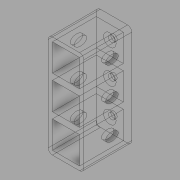
# Autodesk Inventor part: AK-C-C39-Holder
Saved by Autodesk Inventor 2016 (Build 200138000, 138)
## iProperties
Created: 2016-04-02
Part Number: AK-C-C39-Holder
Material: ABS Plastic
Document SubType Name: Modeling
Designer: admin
Density: 1.06 g/cm^3
Appearance: Smooth - White
Author: admin
Autodesk Inventor part; units mm, degrees
ref_plane "YZ Plane" through (0, 0, 0) normal (1, 0, 0) x (0, 1, 0)
ref_plane "XZ Plane" through (0, 0, 0) normal (0, 1, 0) x (-1, 0, 0)
ref_plane "XY Plane" through (0, 0, 0) normal (0, 0, 1) x (1, 0, 0)
derived "AK-C-C39-Main-Board.ipt"
sketch "Sketch2" plane through (0, 0, 0) normal (0, 1, 0) x (-1, 0, 0)
  line L0 (51.25, -29) -> (44.125, -29)
  line L1 (43.25, -29.875) -> (43.25, -31)
  line L2 (43.25, -31) -> (6.5, -31)
  line L3 (6.5, -31) -> (6.5, -29.875)
  line L4 (5.625, -29) -> (-5.625, -29)
  line L5 (-6.5, -29.875) -> (-6.5, -31)
  line L6 (-6.5, -31) -> (-43.25, -31)
  line L7 (-43.25, -31) -> (-43.25, -29.875)
  line L8 (-44.125, -29) -> (-51.25, -29)
  line L9 (-51.25, -29) -> (-53.75, -26.5)
  line L10 (-53.75, -26.5) -> (-53.75, 26.5)
  line L11 (-53.75, 26.5) -> (-51.25, 29)
  line L12 (-51.25, 29) -> (-44.125, 29)
  line L13 (-43.25, 29.875) -> (-43.25, 31)
  line L14 (-43.25, 31) -> (-6.5, 31)
  line L15 (-6.5, 31) -> (-6.5, 29.875)
  line L16 (-5.625, 29) -> (5.625, 29)
  line L17 (6.5, 29.875) -> (6.5, 31)
  line L18 (43.25, 31) -> (43.25, 29.875)
  line L19 (43.25, 31) -> (6.5, 31)
  line L20 (44.125, 29) -> (51.25, 29)
  line L21 (51.25, 29) -> (53.75, 26.5)
  line L22 (53.75, 26.5) -> (53.75, -26.5)
  line L23 (53.75, -26.5) -> (51.25, -29)
  line L24 (44.8, -32.325) -> (5, -32.325)
  line L25 (5, -32.325) -> (5, -29.925)
  line L26 (5, -29.925) -> (3, -29.925)
  line L27 (44.8, -29.925) -> (44.8, -32.325)
  line L28 (46.8, -29.925) -> (44.8, -29.925)
  line L29 (52.8, -29.7756) -> (52.8, -31.925)
  arc A0 (53.6536, -29.4221) -> (52.8, -29.7756) centre (53.3, -29.7756) ccw
  arc A1 (55.3506, -27.225) -> (54.9971, -28.0786) centre (55.3506, -27.725) ccw
  line L30 (55, -17.425) -> (55, -25.225)
  line L31 (0, -6.6233) -> (0, 6.4737) construction
  line L32 (9.5866, 0) -> (-6.7847, 0) construction
  line L33 (57.8, 19.225) -> (57.8, -3.3607)
  line L34 (57.8, -3.3607) -> (55, -7.6074)
  line L35 (55.5, 19.225) -> (57.8, 19.225)
  line L36 (55.5, 29.925) -> (51.9091, 26.3341) construction
  line L37 (25.75, -24.5) -> (12.75, -24.5)
  line L38 (12.75, 24.5) -> (25.75, 24.5)
  line L39 (3.3524, -20) -> (-16.6476, -20)
  line L40 (-16.6476, -20) -> (-16.6476, 20)
  line L41 (-16.6476, 20) -> (3.3524, 20)
  line L42 (3.3524, 20) -> (3.3524, -20)
  line L43 (-23.9878, -15) -> (-31.9878, -15) construction
  line L44 (-31.9878, -15) -> (-31.9878, -7) construction
  line L45 (-31.9878, -7) -> (-23.9878, -7) construction
  line L46 (-23.9878, -7) -> (-23.9878, -15) construction
  line L47 (-34.9878, -15) -> (-42.9878, -15) construction
  line L48 (-42.9878, -15) -> (-42.9878, -7) construction
  line L49 (-42.9878, -7) -> (-34.9878, -7) construction
  line L50 (-34.9878, -7) -> (-34.9878, -15) construction
  line L51 (-23.9878, -4) -> (-31.9878, -4) construction
  line L52 (-31.9878, -4) -> (-31.9878, 4) construction
  line L53 (-31.9878, 4) -> (-23.9878, 4) construction
  line L54 (-23.9878, 4) -> (-23.9878, -4) construction
  line L55 (-34.9878, -4) -> (-42.9878, -4) construction
  line L56 (-42.9878, -4) -> (-42.9878, 4) construction
  line L57 (-42.9878, 4) -> (-34.9878, 4) construction
  line L58 (-34.9878, 4) -> (-34.9878, -4) construction
  line L59 (-23.9878, 7) -> (-31.9878, 7) construction
  line L60 (-31.9878, 7) -> (-31.9878, 15) construction
  line L61 (-31.9878, 15) -> (-23.9878, 15) construction
  line L62 (-23.9878, 15) -> (-23.9878, 7) construction
  line L63 (-34.9878, 7) -> (-42.9878, 7) construction
  line L64 (-42.9878, 7) -> (-42.9878, 15) construction
  line L65 (-42.9878, 15) -> (-34.9878, 15) construction
  line L66 (-34.9878, 15) -> (-34.9878, 7) construction
  line L67 (25.75, -22.5) -> (12.75, -22.5) construction
  line L68 (12.75, -22.5) -> (12.75, -9.5) construction
  line L69 (12.75, -9.5) -> (25.75, -9.5) construction
  line L70 (25.75, -9.5) -> (25.75, -22.5) construction
  line L71 (25.75, -6.5) -> (12.75, -6.5) construction
  line L72 (12.75, -6.5) -> (12.75, 6.5) construction
  line L73 (12.75, 6.5) -> (25.75, 6.5) construction
  line L74 (25.75, 6.5) -> (25.75, -6.5) construction
  line L75 (25.75, 9.5) -> (12.75, 9.5) construction
  line L76 (12.75, 9.5) -> (12.75, 22.5) construction
  line L77 (12.75, 22.5) -> (25.75, 22.5) construction
  line L78 (25.75, 22.5) -> (25.75, 9.5) construction
  line L79 (31.9633, -16) -> (17.7262, -16) construction
  line L80 (31.9633, 16) -> (18.8213, 16) construction
  line L81 (19.25, -23.7063) -> (19.25, 24.6931) construction
  arc A2 (10.75, -22.5) -> (12.75, -24.5) centre (12.75, -22.5) ccw
  arc A3 (25.75, -24.5) -> (27.75, -22.5) centre (25.75, -22.5) ccw
  arc A4 (12.75, 24.5) -> (10.75, 22.5) centre (12.75, 22.5) ccw
  arc A5 (27.75, 22.5) -> (25.75, 24.5) centre (25.75, 22.5) ccw
  line L82 (55, -25.225) -> (-54.9956, -25.225) construction
  line L83 (55.5, 25.225) -> (55.5, 23.225)
  line L84 (57.5, 25.225) -> (55.5, 25.225)
  line L85 (-57.5, 25.225) -> (-55.5, 25.225)
  line L86 (-55.5, 25.225) -> (-55.5, 23.225)
  line L87 (-57.5, -25.225) -> (-55, -25.225)
  line L88 (-55, -25.225) -> (-55, -17.425)
  line L89 (55, -25.225) -> (57.5, -25.225)
  line L90 (55.5, 25.225) -> (-55.5, 25.225) construction
  line L91 (48.25, -2.5) -> (48.25, 2.5)
  line L92 (50, -2.5) -> (50, 2.5)
  line L93 (50, -4) -> (48.25, -4)
  line L94 (50, 4) -> (48.25, 4)
  arc A6 (50, -4) -> (50, -2.5) centre (50, -3.25) ccw
  arc A7 (48.25, -2.5) -> (48.25, -4) centre (48.25, -3.25) ccw
  arc A8 (50, 2.5) -> (50, 4) centre (50, 3.25) ccw
  arc A9 (48.25, 4) -> (48.25, 2.5) centre (48.25, 3.25) ccw
  line L95 (-37.75, -2.5) -> (-37.75, 2.5)
  line L96 (-39.5, 4) -> (-37.75, 4)
  line L97 (-39.5, 2.5) -> (-39.5, -2.5)
  line L98 (-39.5, -4) -> (-37.75, -4)
  arc A10 (-37.75, -4) -> (-37.75, -2.5) centre (-37.75, -3.25) ccw
  arc A11 (-39.5, -2.5) -> (-39.5, -4) centre (-39.5, -3.25) ccw
  arc A12 (-37.75, 2.5) -> (-37.75, 4) centre (-37.75, 3.25) ccw
  arc A13 (-39.5, 4) -> (-39.5, 2.5) centre (-39.5, 3.25) ccw
  line L99 (48.75, -27) -> (40.5, -27)
  line L100 (38.75, -27) -> (38.75, -25.25)
  line L101 (40.5, -25.25) -> (48.75, -25.25)
  line L102 (1.75, -27) -> (-8.25, -27)
  line L103 (-8.25, -25.25) -> (1.75, -25.25)
  line L104 (-40, -27) -> (-48.25, -27)
  line L105 (-48.25, -25.25) -> (-40, -25.25)
  line L106 (-48.25, 25.25) -> (-40, 25.25)
  line L107 (-40, 27) -> (-48.25, 27)
  line L108 (1.75, 25.25) -> (-8.25, 25.25)
  line L109 (-8.25, 27) -> (1.75, 27)
  line L110 (48.75, 25.25) -> (40.25, 25.25)
  line L111 (38.75, 25.25) -> (38.75, 27)
  line L112 (40.25, 27) -> (48.75, 27)
  arc A14 (38.75, -27) -> (40.5, -27) centre (39.625, -27) ccw
  arc A15 (40.5, -25.25) -> (38.75, -25.25) centre (39.625, -25.25) ccw
  arc A16 (38.75, 25.25) -> (40.25, 25.25) centre (39.5, 25.25) ccw
  arc A17 (40.25, 27) -> (38.75, 27) centre (39.5, 27) ccw
  line L113 (27.75, 22.5) -> (27.75, -22.5)
  line L114 (-34.9878, 7) -> (-42.9878, 15) construction
  line L115 (-31.9878, 7) -> (-23.9878, 15) construction
  line L116 (-31.9878, -7) -> (-23.9878, -15) construction
  line L117 (-34.9878, -7) -> (-42.9878, -15) construction
  line L118 (10.75, 7.999) -> (10.75, 8)
  line L119 (10.75, -22.5) -> (10.75, 22.5)
  arc A18 (48.75, 25.25) -> (48.75, 27) centre (48.75, 26.125) ccw
  arc A19 (-8.25, 27) -> (-8.25, 25.25) centre (-8.25, 26.125) ccw
  arc A20 (-48.25, 27) -> (-48.25, 25.25) centre (-48.25, 26.125) ccw
  arc A21 (48.75, -27) -> (48.75, -25.25) centre (48.75, -26.125) ccw
  arc A22 (-8.25, -25.25) -> (-8.25, -27) centre (-8.25, -26.125) ccw
  arc A23 (-48.25, -25.25) -> (-48.25, -27) centre (-48.25, -26.125) ccw
  line L120 (31, 25) -> (29.25, 25)
  line L121 (31, 23.5) -> (31, 20)
  line L122 (29.25, 20) -> (29.25, 23.5)
  arc A24 (31, 23.5) -> (31, 25) centre (31, 24.25) ccw
  arc A25 (29.25, 25) -> (29.25, 23.5) centre (29.25, 24.25) ccw
  arc A26 (29.25, 20) -> (31, 20) centre (30.125, 20) ccw
  line L123 (29.25, -20) -> (29.25, -23.25)
  line L124 (29.25, -25) -> (31, -25)
  line L125 (31, -23.25) -> (31, -20)
  arc A27 (31, -25) -> (31, -23.25) centre (31, -24.125) ccw
  arc A28 (29.25, -23.25) -> (29.25, -25) centre (29.25, -24.125) ccw
  arc A29 (31, -20) -> (29.25, -20) centre (30.125, -20) ccw
  line L126 (9.25, 25) -> (7.5, 25)
  line L127 (7.5, 23.5) -> (7.5, 20)
  line L128 (9.25, 20) -> (9.25, 23.5)
  line L129 (7.5, -20) -> (7.5, -23.25)
  line L130 (7.5, -25) -> (9.25, -25)
  line L131 (9.25, -23.25) -> (9.25, -20)
  arc A30 (9.25, -20) -> (7.5, -20) centre (8.375, -20) ccw
  arc A31 (9.25, -25) -> (9.25, -23.25) centre (9.25, -24.125) ccw
  arc A32 (7.5, -23.25) -> (7.5, -25) centre (7.5, -24.125) ccw
  arc A33 (7.5, 20) -> (9.25, 20) centre (8.375, 20) ccw
  arc A34 (9.25, 23.5) -> (9.25, 25) centre (9.25, 24.25) ccw
  arc A35 (7.5, 25) -> (7.5, 23.5) centre (7.5, 24.25) ccw
  line L132 (29.25, 4) -> (29.25, -4)
  line L133 (31, -4) -> (31, 4)
  line L134 (7.5, 4) -> (7.5, -4)
  line L135 (9.25, -4) -> (9.25, 4)
  arc A36 (31, 4) -> (29.25, 4) centre (30.125, 4) ccw
  arc A37 (29.25, -4) -> (31, -4) centre (30.125, -4) ccw
  arc A38 (9.25, 4) -> (7.5, 4) centre (8.375, 4) ccw
  arc A39 (7.5, -4) -> (9.25, -4) centre (8.375, -4) ccw
  line L136 (-14.75, 30.3253) -> (-31.75, 30.3253) construction
  line L137 (-31.75, 30.3253) -> (-31.75, 22.4164) construction
  line L138 (-31.75, 22.4164) -> (-14.75, 22.4164) construction
  line L139 (-14.75, 22.4164) -> (-14.75, 30.3253) construction
  line L140 (-23.25, 29.9722) -> (-23.25, 20.9797) construction
  arc A40 (6.5, -29.875) -> (5.625, -29) centre (5.625, -29.875) ccw
  arc A41 (-5.625, -29) -> (-6.5, -29.875) centre (-5.625, -29.875) ccw
  arc A42 (-43.25, -29.875) -> (-44.125, -29) centre (-44.125, -29.875) ccw
  arc A43 (-44.125, 29) -> (-43.25, 29.875) centre (-44.125, 29.875) ccw
  arc A44 (-6.5, 29.875) -> (-5.625, 29) centre (-5.625, 29.875) ccw
  arc A45 (5.625, 29) -> (6.5, 29.875) centre (5.625, 29.875) ccw
  arc A46 (43.25, 29.875) -> (44.125, 29) centre (44.125, 29.875) ccw
  arc A47 (44.125, -29) -> (43.25, -29.875) centre (44.125, -29.875) ccw
  line L141 (57.5, 27.225) -> (57.5, 25.225)
  line L142 (-57.5, 27.225) -> (-57.5, 25.225)
  arc A48 (1.75, 25.25) -> (1.75, 27) centre (1.75, 26.125) ccw
  arc A49 (1.75, -27) -> (1.75, -25.25) centre (1.75, -26.125) ccw
  arc A50 (-38.25, 27) -> (-40, 27) centre (-39.125, 27) ccw
  arc A51 (-40, 25.25) -> (-38.25, 25.25) centre (-39.125, 25.25) ccw
  line L143 (-38.25, 27) -> (-38.25, 25.25)
  arc A52 (-38.25, -25.25) -> (-40, -25.25) centre (-39.125, -25.25) ccw
  arc A53 (-40, -27) -> (-38.25, -27) centre (-39.125, -27) ccw
  line L144 (-38.25, -25.25) -> (-38.25, -27)
  line L145 (-60, -16.775) -> (-60, 29.925)
  point P0 (53.75, -25.225)
  point P1 (25.75, -16)
  point P2 (25.75, 16)
  point P3 (19.25, -22.5)
  point P4 (19.25, -24.5)
  point P5 (27.75, 0)
  point P6 (10.75, 0)
  point P7 (-23.25, 30.3253)
  point P8 (-23.25, 18)
  point P9 (-23.25, -18)
  point P10 (-53.75, -25.225)
sketch "Sketch3" plane through (0, 0, 0) normal (0, 1, 0) x (-1, 0, 0)
  line L0 (55, -25.225) -> (-54.9956, -25.225) construction
  line L1 (55.5, 25.225) -> (-55.5, 25.225) construction
  arc A0 (27.75, 22.5) -> (25.75, 24.5) centre (25.75, 22.5) ccw projected
  line L2 (12.75, 24.5) -> (25.75, 24.5) projected
  arc A1 (12.75, 24.5) -> (10.75, 22.5) centre (12.75, 22.5) ccw projected
  line L3 (10.75, -22.5) -> (10.75, 22.5) projected
  arc A2 (10.75, -22.5) -> (12.75, -24.5) centre (12.75, -22.5) ccw projected
  line L4 (25.75, -24.5) -> (12.75, -24.5) projected
  arc A3 (25.75, -24.5) -> (27.75, -22.5) centre (25.75, -22.5) ccw projected
  line L5 (27.75, 22.5) -> (27.75, -22.5) projected
  point P0 (0, 0)
extrude "Extrusion1" add sketch "Sketch3" along normal blind 4.6
sketch "Sketch4" plane through (0, 4.6, 0) normal (0, 1, 0) x (1, 0, 0)
  line L0 (-55, 25.225) -> (54.9956, 25.225) construction
  line L1 (-55.5, -25.225) -> (55.5, -25.225) construction
  line L2 (-27.75, -22.5) -> (-27.75, 22.5) projected
  arc A0 (-27.75, -22.5) -> (-25.75, -24.5) centre (-25.75, -22.5) ccw projected
  line L3 (-12.75, -24.5) -> (-25.75, -24.5) projected
  arc A1 (-12.75, -24.5) -> (-10.75, -22.5) centre (-12.75, -22.5) ccw projected
  line L4 (-10.75, 22.5) -> (-10.75, -22.5) projected
  arc A2 (-10.75, 22.5) -> (-12.75, 24.5) centre (-12.75, 22.5) ccw projected
  line L5 (-12.75, 24.5) -> (-25.75, 24.5) projected
  arc A3 (-25.75, 24.5) -> (-27.75, 22.5) centre (-25.75, 22.5) ccw projected
  point P0 (0, 0)
extrude "Extrusion2" add sketch "Sketch4" along normal blind 18.4
sketch "Sketch6" plane through (0, 0, 0) normal (0, -1, 0) x (1, 0, 0)
  line L0 (-25.75, 22.5) -> (-25.75, 9.5) projected
  line L1 (-12.75, 22.5) -> (-25.75, 22.5) projected
  line L2 (-12.75, 9.5) -> (-12.75, 22.5) projected
  line L3 (-25.75, 9.5) -> (-12.75, 9.5) projected
  line L4 (-12.75, 6.5) -> (-25.75, 6.5) projected
  line L5 (-25.75, 6.5) -> (-25.75, -6.5) projected
  line L6 (-25.75, -6.5) -> (-12.75, -6.5) projected
  line L7 (-12.75, -6.5) -> (-12.75, 6.5) projected
  line L8 (-12.75, -9.5) -> (-25.75, -9.5) projected
  line L9 (-25.75, -9.5) -> (-25.75, -22.5) projected
  line L10 (-25.75, -22.5) -> (-12.75, -22.5) projected
  line L11 (-12.75, -22.5) -> (-12.75, -9.5) projected
  point P0 (0, 0)
extrude "Extrusion4" cut sketch "Sketch6" against normal blind 21
sketch "Sketch10" plane through (-10.75, 0, 22.5) normal (1, 0, 0) x (0, 0, -1)
  ellipse E0 centre (38.5, 13.5) end of major axis (36.5, 13.5) minor radius 3
  ellipse E1 centre (22.5, 13.5) end of major axis (20.5, 13.5) minor radius 3
  ellipse E2 centre (6.5, 13.5) end of major axis (4.5, 13.5) minor radius 3
  line L0 (45, 23) -> (0, 23)
  line L1 (32, 0) -> (45, 0)
  line L2 (16, 0) -> (29, 0)
  line L3 (0, 0) -> (13, 0)
  point P0 (38.5, 0)
  point P1 (22.5, 0)
  point P2 (6.5, 0)
  dimension "d34" = 3
  dimension "d35" = 2
  dimension "d36" = 3
  dimension "d37" = 2
  dimension "d38" = 3
  dimension "d39" = 2
  dimension "d41" = 9.5
  constraints: 8 end point, 3 midpoint, 3 vertical alignment, 2 horizontal alignment, 6 other
  measures "d41" distance from line of L0 point (6.5, 13.5)
extrude "Extrusion6" cut sketch "Sketch10" against normal through all
sketch "Sketch9" plane through (0, 21, 0) normal (0, -1, 0) x (1, 0, 0)
  line L0 (-31.9633, 16) -> (-18.8213, 16) construction
  line L1 (-19.25, -23.7063) -> (-19.25, 24.6931) construction
  line L2 (-9.5866, 0) -> (6.7847, 0) construction
  line L3 (-31.9633, -16) -> (-17.7262, -16) construction
  point P0 (0, 0)
  point P1 (-19.25, 16)
  point P2 (-19.25, 0)
  point P3 (-19.25, -16)
  constraints: 6 point on line
hole "Hole1" at (-19.25, 21, 16) at (-19.25, 21, 0) at (-19.25, 21, -16) direction (0, 1, 0) diameter 3 end through all countersink diameter 6 countersink angle 120
sketch "Sketch5" plane through (0, 23, 0) normal (0, 1, 0) x (1, 0, 0)
  arc A0 (-32.45, -12.75) -> (-32.45, -19.25) centre (-32.45, -16) ccw
  arc A1 (-32.45, 19.25) -> (-32.45, 12.75) centre (-32.45, 16) ccw
  arc A2 (-6.95, -19.25) -> (-6.95, -12.75) centre (-6.95, -16) ccw
  arc A3 (-6.95, 12.75) -> (-6.95, 19.25) centre (-6.95, 16) ccw
  line L0 (-27.2, -24.5) -> (-12.2, -24.5) projected
  arc A4 (-29.2, -22.5) -> (-27.2, -24.5) centre (-27.2, -22.5) ccw projected
  line L1 (-29.2, 22.5) -> (-29.2, -22.5) projected
  arc A5 (-27.2, 24.5) -> (-29.2, 22.5) centre (-27.2, 22.5) ccw projected
  line L2 (-12.2, 24.5) -> (-27.2, 24.5) projected
  arc A6 (-10.2, 22.5) -> (-12.2, 24.5) centre (-12.2, 22.5) ccw projected
  line L3 (-10.2, -22.5) -> (-10.2, 22.5) projected
  arc A7 (-12.2, -24.5) -> (-10.2, -22.5) centre (-12.2, -22.5) ccw projected
  arc A8 (-32.45, 19.25) -> (-29.2, 22.5) centre (-32.45, 22.5) ccw
  arc A9 (-29.2, 9.5) -> (-32.45, 12.75) centre (-32.45, 9.5) ccw
  arc A10 (-6.95, 12.75) -> (-10.2, 9.5) centre (-6.95, 9.5) ccw
  arc A11 (-32.45, -12.75) -> (-29.2, -9.5) centre (-32.45, -9.5) ccw
  arc A12 (-29.2, -22.5) -> (-32.45, -19.25) centre (-32.45, -22.5) ccw
  arc A13 (-10.2, -9.5) -> (-6.95, -12.75) centre (-6.95, -9.5) ccw
  arc A14 (-6.95, -19.25) -> (-10.2, -22.5) centre (-6.95, -22.5) ccw
  arc A15 (-10.2, 22.5) -> (-6.95, 19.25) centre (-6.95, 22.5) ccw
  line L4 (-31.9633, -16) -> (-18.8213, -16) construction
  point P0 (0, 0)
  constraints: 27 point on circle, 20 tangent, 12 centre point, 10 equal radius, 5 point on line, 4 horizontal alignment, 1 end point, 1 vertical alignment
body "Solid1"
